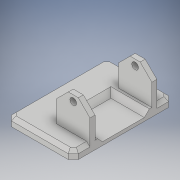
# Autodesk Inventor part: Pezotta
Saved by Autodesk Inventor 2019.1 (Build 231200000, 200)
## iProperties
Created: 2019-07-25
Part Number: Pezotta
Material: Genérico
Document SubType Name: Modeling
Designer: IEEE UFABC
Density: 1 g/cm^3
Appearance: Padrão
Author: IEEE UFABC
Autodesk Inventor part; units mm, degrees
ref_plane "YZ Plane" through (0, 0, 0) normal (1, 0, 0) x (0, 1, 0)
ref_plane "XZ Plane" through (0, 0, 0) normal (0, 1, 0) x (-1, 0, 0)
ref_plane "XY Plane" through (0, 0, 0) normal (0, 0, 1) x (1, 0, 0)
sketch "Esboço1" plane through (0, 0, 0) normal (0, 1, 0) x (-1, 0, 0)
  line L0 (0, 0) -> (40, 0)
  line L1 (40, 0) -> (40, -60)
  line L2 (40, -60) -> (0, -60)
  line L3 (0, -60) -> (0, 0)
  dimension "d0" = 40
  dimension "d1" = 60
  constraints: 8 end point, 2 parallel, 1 horizontal, 1 perpendicular
  measures "d0" distance of L1.end L2.end
  measures "d1" distance of L0.end L1.end
extrude "Extrusão1" add sketch "Esboço1" along normal blind 5
chamfer "Chanfro1" distance 3 angle 45 4 edges at (0, 2.5, 0) (-40, 2.5, 0) (0, 2.5, -60) (-40, 2.5, -60)
sketch "Esboço2" plane through (0, 5, 0) normal (0, 1, 0) x (1, 0, 0)
  line L0 (-3, 60) -> (-37, 60) construction
  line L1 (-20, 60) -> (-20, 0) construction
  line L2 (-20, 30) -> (0, 30) construction
  line L3 (-3, 30) -> (-3, 50) construction
  line L4 (-3, 30) -> (-3, 10) construction
  line L5 (0, 3) -> (0, 57) projected
  line L6 (0, 10) -> (-20, 10)
  line L7 (-20, 10) -> (-20, 13)
  line L8 (-20, 13) -> (0, 13)
  line L9 (0, 13) -> (0, 10)
  line L10 (0, 50) -> (-20, 50)
  line L11 (-20, 50) -> (-20, 47)
  line L12 (-20, 47) -> (0, 47)
  line L13 (0, 47) -> (0, 50)
  point P0 (0, 0)
  dimension "d7" = 20
  dimension "d8" = 20
  dimension "d9" = 3
  dimension "d10" = 3
  constraints: 24 end point, 5 point on line, 4 parallel, 3 horizontal, 3 vertical, 2 midpoint, 2 perpendicular
  measures "d7" distance of L3.start L3.end
  measures "d8" distance of L3.start L4.end
  measures "d9" distance of L6.end L7.end
  measures "d10" distance of L11.end L10.end
extrude "Extrusão2" add sketch "Esboço2" along normal blind 20
chamfer "Chanfro2" distance 7 angle 45 4 edges at (-20, 25, -11.5) (0, 25, -11.5) (0, 25, -48.5) (-20, 25, -48.5)
sketch "Esboço3" plane through (0, 5, -13) normal (0, 0, -1) x (-1, 0, 0)
  line L0 (0, 13) -> (20, 13) construction
  line L1 (0, 13) -> (20, 13) construction
  line L2 (10, 13) -> (10, 20) construction
  line L3 (13, 20) -> (7, 20) construction
  circle A0 centre (10, 16.5) radius 2
  point P0 (0, -5)
  dimension "d16" = 4
  constraints: 6 end point, 3 midpoint, 1 centre point, 1 collinear, 1 horizontal
  measures "d16" diameter of A0
extrude "Extrusão3" cut sketch "Esboço3" against normal blind 20
sketch "Esboço4" plane through (-20, 5, -47) normal (0, 0, 1) x (1, 0, 0)
  line L0 (0, 0) -> (0, 13) construction
  line L1 (20, 0) -> (20, 13) construction
  line L2 (0, 13) -> (20, 13) construction
  line L3 (20, 13) -> (10, 13) construction
  line L4 (10, 13) -> (10, 20) construction
  line L5 (13, 20) -> (7, 20) construction
  circle A0 centre (10, 16.5) radius 2
  point P0 (20, -5)
  dimension "d19" = 4
  constraints: 6 end point, 3 midpoint, 1 centre point, 1 horizontal
  measures "d19" diameter of A0
extrude "Extrusão4" cut sketch "Esboço4" against normal blind 666
chamfer "Chanfro3" distance 2 angle 45 9 edges at (-20, 5, -60) (-38.5, 5, -58.5) (-40, 5, -30) (-38.5, 5, -1.5) (-20, 5, 0) (-1.5, 5, -1.5) (0, 5, -6.5) (0, 5, -53.5) (-1.5, 5, -58.5)
sketch "Esboço5" plane through (0, 5, 0) normal (0, 1, 0) x (1, 0, 0)
  line L0 (0, 57) -> (0, 3) projected
  line L1 (0, 17.5) -> (-20, 17.5)
  line L2 (-20, 17.5) -> (-20, 42.5)
  line L3 (-20, 42.5) -> (0, 42.5)
  line L4 (0, 42.5) -> (0, 17.5)
  line L5 (-7, 13) -> (-13, 13) projected
  point P0 (0, 0)
  dimension "d25" = 20
  dimension "d26" = 25
  dimension "d27" = 4.5
  constraints: 8 end point, 2 parallel, 1 horizontal, 1 perpendicular, 1 point on line
  measures "d25" distance of L2.end L3.end
  measures "d26" distance of L1.end L2.end
  measures "d27" distance between parallel lines of L5 L1
extrude "Extrusão5" cut sketch "Esboço5" against normal blind 3
chamfer "Chanfro4" distance 3 angle 45 3 edges at (-20, 5, -30) (-10, 5, -42.5) (-10, 5, -17.5)
